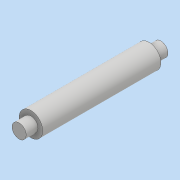
# Autodesk Inventor part: P9
Saved by Autodesk Inventor 2017 (Build 210142000, 142)
## iProperties
Part Number: P9
Material: 一般
Document SubType Name: Modeling
Designer: d8910
Density: 1 g/cm^3
Appearance: 預設
Author: d8910
Autodesk Inventor part; units mm, degrees
ref_plane "YZ Plane" through (0, 0, 0) normal (1, 0, 0) x (0, 1, 0)
ref_plane "XZ Plane" through (0, 0, 0) normal (0, 1, 0) x (-1, 0, 0)
ref_plane "XY Plane" through (0, 0, 0) normal (0, 0, 1) x (1, 0, 0)
sketch "草圖1" plane through (0, 0, 0) normal (0, 0, 1) x (1, 0, 0)
  line L0 (0, 50) -> (10, 50)
  line L1 (10, 50) -> (10, -50)
  line L2 (10, -50) -> (0, -50)
  line L3 (0, -50) -> (0, 50)
  line L4 (0, 50) -> (6, 50)
  line L5 (6, 50) -> (6, 60)
  line L6 (6, 60) -> (0, 60)
  line L7 (0, 60) -> (0, 50)
  line L8 (0, -50) -> (6, -50)
  line L9 (6, -50) -> (6, -60)
  line L10 (6, -60) -> (0, -60)
  line L11 (0, -60) -> (0, -50)
  point P0 (0, 0)
  point P1 (10, 0)
  dimension "d0" = 10
  dimension "d1" = 6
  dimension "d2" = 6
  dimension "d3" = 120
  dimension "d4" = 100
  dimension "d5" = 10
  constraints: 24 end point, 6 parallel, 4 vertical alignment, 3 horizontal, 3 perpendicular, 1 horizontal alignment, 1 midpoint
  measures "d0" distance between parallel lines of L3 L1
  measures "d1" distance between parallel lines of L7 L5
  measures "d2" distance of L9.end L10.end
  measures "d3" distance between parallel lines of L10 L6
  measures "d4" distance of L0.end L1.end
  measures "d5" distance of L8.end L9.end
revolve "迴轉1" add sketch "草圖1" angle 360 about axis through (0, -50, 0) along (0, 1, 0)
